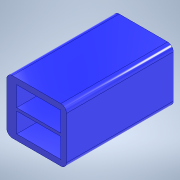
# Autodesk Inventor part: Electronics Mount
Saved by Autodesk Inventor 2022 (Build 260153000, 153)
## iProperties
Created: 2022-08-13
Part Number: Electronics Mount
Material: Generic
Document SubType Name: Modeling
Designer: Nick
Density: 0.880757 g/cm^3
Appearance: Blue - Wall Paint - Glossy
Mass: 39 g
Surface Area: 312.32 cm^2
Volume: 44.2801 cm^3
Author: Nick
Autodesk Inventor part; units mm, degrees
ref_plane "YZ Plane" through (0, 0, 0) normal (1, 0, 0) x (0, 1, 0)
ref_plane "XZ Plane" through (0, 0, 0) normal (0, 1, 0) x (-1, 0, 0)
sketch "Sketch1" plane through (0, 0, 0) normal (0, 0, 1) x (1, 0, 0)
  line L0 (0, 0) -> (31, 0)
  line L1 (31, 0) -> (31, 4)
  line L2 (31, 4) -> (0, 4)
  line L3 (0, 4) -> (0, 0)
  line L4 (0, 18) -> (31, 18)
  line L5 (31, 18) -> (31, 20)
  line L6 (31, 20) -> (0, 20)
  line L7 (0, 20) -> (0, 18)
  line L8 (0, 34) -> (31, 34)
  line L9 (31, 34) -> (31, 38)
  line L10 (31, 38) -> (0, 38)
  line L11 (0, 38) -> (0, 34)
  line L12 (-7, 38) -> (0, 38)
  line L13 (0, 38) -> (0, 0)
  line L14 (0, 0) -> (-7, 0)
  line L15 (-7, 0) -> (-7, 38)
  line L16 (35, 38) -> (31, 38)
  line L17 (31, 38) -> (31, 0)
  line L18 (31, 0) -> (35, 0)
  line L19 (35, 0) -> (35, 38)
  point P0 (0, 4)
  point P1 (0, 18)
  point P2 (0, 20)
  point P3 (0, 34)
  dimension "d1" = 31
  dimension "d3" = 14
  dimension "d4" = 14
  dimension "d7" = 4
  dimension "d25" = 2
  dimension "d26" = 7
  dimension "d27" = 4
  constraints: 40 end point, 10 parallel, 5 collinear, 5 horizontal, 5 perpendicular, 2 point on line
  measures "d1" distance of L4.start L4.end
  measures "d3" distance between parallel lines of L6 L8
  measures "d4" distance between parallel lines of L2 L4
  measures "d7" distance of L8.end L9.end
  measures "d25" distance of L4.end L5.end
  measures "d26" distance of L12.start L12.end
  measures "d27" distance of L0.end L18.end
extrude "Extrusion1" add sketch "Sketch1" along normal blind 75 contours L3 L2 L1 L0 | L14 L15 L12 L11 L13 L7 L3 | L1 L17 L5 L9 L16 L19 L18 | L7 L6 L5 L4 | L10 L9 L8 L11
ref_plane "Work Plane5" through (-6.2, 0, 0) normal (-1, 0, 0) x (0, 0, 1)
sketch "Sketch4" plane through (-7, 0, 0) normal (-1, 0, 0) x (0, 0, 1)
  circle A0 centre (19, 19) radius 16.002
  circle A1 centre (56, 19) radius 16.002
  line L0 (75, 38) -> (75, 0) projected
  line L1 (0, 38) -> (0, 0) projected
  line L2 (56, 35.002) -> (72.002, 35.002)
  line L3 (72.002, 35.002) -> (72.002, 2.998)
  line L4 (72.002, 2.998) -> (56, 2.998)
  line L5 (19, 35.002) -> (35.002, 35.002)
  line L6 (35.002, 35.002) -> (35.002, 2.998)
  line L7 (35.002, 2.998) -> (19, 2.998)
  point P0 (0, 19)
  point P1 (35.002, 19)
  point P2 (72.002, 19)
  dimension "d28" = 32.004
  dimension "d29" = 32.004
  dimension "d32" = 19
  dimension "d33" = 19
  constraints: 12 end point, 6 tangent, 4 horizontal, 4 point on circle, 2 centre point, 2 horizontal alignment, 2 vertical, 1 midpoint
  measures "d28" diameter of A0
  measures "d29" diameter of A1
  measures "d32" distance from line of L1 A0.centre
  measures "d33" distance from line of L0 A1.centre
extrude "Extrusion4" cut sketch "Sketch4" against normal blind 5.08 from surface at -0.8
fillet "Fillet2" radius 4 4 edges at (-7, 38, 37.5) (35, 38, 37.5) (35, 0, 37.5) (-7, 0, 37.5)
equation "\"d3\" = d4"
body "Solid1"
